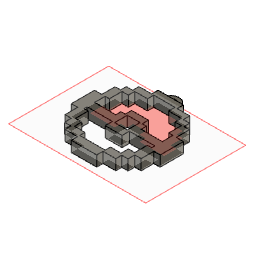
keychain (Autodesk Fusion 360 design; units mm, degrees)
Autodesk Fusion 360 part; units mm, degrees
sketch "Sketch1" plane through (0, 0, 0) normal (0, 0, 1) x (1, 0, 0)
sketch "Sketch2" plane through (0, 0, 0) normal (0, 0, 1) x (1, 0, 0)
  line L0 (12, 30) -> (12, 19)
  line L1 (12, 19) -> (15, 19)
  line L2 (15, 19) -> (15, 13)
  line L3 (15, 13) -> (18, 13)
  line L4 (18, 13) -> (18, 9.8247)
  line L5 (18, 9.8247) -> (21, 9.8247)
  line L6 (21, 9.8247) -> (21, 7)
  line L7 (21, 7) -> (27, 7)
  line L8 (27, 7) -> (27, 4)
  line L9 (12, 30) -> (15.3965, 30)
  line L10 (15.3965, 30) -> (15.3965, 36.3062)
  line L11 (15.3965, 36.3062) -> (18, 36.3062)
  line L12 (18, 36.3062) -> (18, 39)
  line L13 (18, 39) -> (21, 39)
  line L14 (21, 39) -> (21, 42)
  line L15 (21, 42) -> (27, 42)
  line L16 (27, 42) -> (27, 45)
  line L17 (45, 42) -> (39, 42)
  line L18 (39, 42) -> (39, 45)
  line L19 (45, 39) -> (45, 42)
  line L20 (48, 39) -> (45, 39)
  line L21 (48, 36.3062) -> (48, 39)
  line L22 (50.6035, 36.3062) -> (48, 36.3062)
  line L23 (50.6035, 30) -> (50.6035, 36.3062)
  line L24 (54, 30) -> (50.6035, 30)
  line L25 (54, 30) -> (54, 19)
  line L26 (54, 19) -> (51, 19)
  line L27 (51, 19) -> (51, 13)
  line L28 (51, 13) -> (48, 13)
  line L29 (48, 13) -> (48, 9.8247)
  line L30 (48, 9.8247) -> (45, 9.8247)
  line L31 (45, 9.8247) -> (45, 7)
  line L32 (45, 7) -> (39, 7)
  line L33 (39, 7) -> (39, 4)
  line L34 (27, 45) -> (39, 45)
  line L35 (27, 4) -> (39, 4)
  line L36 (30, 27.5) -> (30, 21.5)
  line L37 (30, 21.5) -> (33, 21.5)
  line L38 (30, 27.5) -> (33, 27.5)
  line L39 (36, 27.5) -> (33, 27.5)
  line L40 (36, 27.5) -> (36, 21.5)
  line L41 (36, 21.5) -> (33, 21.5)
  line L42 (17, 20) -> (19, 20)
  line L43 (19, 20) -> (19, 14)
  line L44 (19, 14) -> (22, 14)
  line L45 (22, 14) -> (22, 10.5215)
  line L46 (22, 10.5215) -> (27, 10.5215)
  line L47 (27, 10.5215) -> (27, 8)
  line L48 (27, 8) -> (33, 8)
  line L49 (17, 20) -> (17, 21.4527)
  line L50 (17, 21.4527) -> (27, 21.4527)
  line L51 (27, 21.4527) -> (29, 21.4527)
  line L52 (29, 21.4527) -> (29, 18)
  line L53 (29, 18) -> (33, 18)
  line L54 (17, 30) -> (17, 25)
  line L55 (17, 25) -> (27, 25)
  line L56 (27, 25) -> (27, 27.5)
  line L57 (27, 27.5) -> (29, 27.5)
  line L58 (29, 27.5) -> (29, 30.5)
  line L59 (29, 30.5) -> (33, 30.5)
  line L60 (17, 30) -> (19, 30)
  line L61 (19, 30) -> (19, 36)
  line L62 (19, 36) -> (22, 36)
  line L63 (22, 36) -> (22, 39)
  line L64 (22, 39) -> (28, 39)
  line L65 (28, 39) -> (28, 42)
  line L66 (28, 42) -> (33, 42)
  line L67 (38, 42) -> (33, 42)
  line L68 (38, 39) -> (38, 42)
  line L69 (44, 39) -> (38, 39)
  line L70 (44, 36) -> (44, 39)
  line L71 (47, 36) -> (44, 36)
  line L72 (47, 30) -> (47, 36)
  line L73 (49, 30) -> (47, 30)
  line L74 (49, 30) -> (49, 25)
  line L75 (49, 25) -> (39, 25)
  line L76 (39, 25) -> (39, 27.5)
  line L77 (37, 27.5) -> (37, 30.5)
  line L78 (37, 30.5) -> (33, 30.5)
  line L79 (49, 21.4527) -> (39, 21.4527)
  line L80 (39, 21.4527) -> (37, 21.4527)
  line L81 (37, 21.4527) -> (37, 18)
  line L82 (37, 18) -> (33, 18)
  line L83 (49, 20) -> (47, 20)
  line L84 (47, 20) -> (47, 14)
  line L85 (47, 14) -> (44, 14)
  line L86 (44, 14) -> (44, 10.5215)
  line L87 (44, 10.5215) -> (39, 10.5215)
  line L88 (39, 10.5215) -> (39, 8)
  line L89 (39, 8) -> (33, 8)
  line L90 (49, 20) -> (49, 21.4527)
  line L91 (39, 27.5) -> (37, 27.5)
  constraint vertical L0
  constraint perpendicular L0 L1
  constraint perpendicular L1 L2
  constraint perpendicular L0 L3
  constraint perpendicular L3 L4
  constraint perpendicular L4 L5
  constraint perpendicular L5 L6
  constraint perpendicular L6 L7
  constraint perpendicular L7 L8
  constraint perpendicular L0 L9
  constraint perpendicular L9 L10
  constraint perpendicular L10 L11
  constraint perpendicular L11 L12
  constraint perpendicular L12 L13
  constraint perpendicular L13 L14
  constraint perpendicular L14 L15
  constraint perpendicular L13 L16
  constraint vertical L36
  constraint perpendicular L2 L42
  constraint perpendicular L42 L43
  constraint perpendicular L2 L44
  constraint perpendicular L42 L45
  constraint perpendicular L45 L46
  constraint perpendicular L46 L47
  constraint perpendicular L42 L49
  constraint perpendicular L49 L50
  constraint perpendicular L36 L51
  constraint perpendicular L51 L52
  constraint perpendicular L9 L54
  constraint perpendicular L54 L55
  constraint perpendicular L55 L56
  constraint perpendicular L36 L57
  constraint perpendicular L38 L58
  constraint perpendicular L54 L60
  constraint perpendicular L60 L61
  constraint perpendicular L61 L62
  constraint perpendicular L62 L63
  constraint perpendicular L61 L64
  constraint perpendicular L64 L65
sketch "Sketch3" plane through (0, 0, 0) normal (0, 0, 1) x (1, 0, 0)
  circle A0 centre (33, 45) radius 2.2361
  circle A1 centre (33, 45) radius 3.9672
  line L0 (29.0331, 45.043) -> (36.9669, 45.043)
  constraint concentric A0 A1
  constraint coincident A1 L0.start
  constraint coincident A1 L0.end
  constraint horizontal L0
extrude "Extrude1" add sketch "Sketch2" along normal blind 5 makes body 1
extrude "Extrude2" add sketch "Sketch3" along normal blind 3 separate body contours A0 A1 L0 picked at (36.3731, 45.2386) makes body 2
